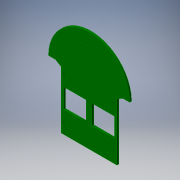
# Autodesk Inventor part: Micromouse1.2.kicad_pcb
Saved by Autodesk Inventor 2016 (Build 200138000, 138)
## iProperties
Created: 2017-09-20
Part Number: Micromouse1.2.kicad_pcb
Material: Generic
Document SubType Name: Modeling
Designer: test
Density: 1 g/cm^3
Appearance: Board Outline
Author: test
Autodesk Inventor part; units mm, degrees
ref_plane "YZ Plane" through (0, 0, 0) normal (1, 0, 0) x (0, 1, 0)
ref_plane "XZ Plane" through (0, 0, 0) normal (0, 1, 0) x (-1, 0, 0)
ref_plane "XY Plane" through (0, 0, 0) normal (0, 0, 1) x (1, 0, 0)
sketch "Sketch1" plane through (0, 0, 0) normal (0, 0, 1) x (1, 0, 0)
  line L0 (83.5624, -61.7466) -> (89.5624, -61.7716)
  line L1 (89.5624, -61.7716) -> (94.5924, -64.7466)
  line L2 (94.5924, -64.7466) -> (94.5924, -114.4666)
  line L3 (94.5924, -114.4666) -> (142.9124, -114.4666)
  line L4 (142.9124, -114.4666) -> (142.9124, -64.7466)
  line L5 (142.9124, -64.7466) -> (148.0124, -61.7466)
  line L6 (148.0124, -61.7466) -> (153.9624, -61.7466)
  arc A0 (153.9624, -61.7466) -> (83.5624, -61.7466) centre (118.7624, -61.7466) ccw
  line L7 (96.775, -95.75) -> (96.775, -78.75)
  line L8 (96.775, -78.75) -> (116.275, -78.75)
  line L9 (116.275, -78.75) -> (116.275, -95.75)
  line L10 (116.275, -95.75) -> (96.775, -95.75)
  line L11 (121.25, -95.775) -> (121.25, -78.775)
  line L12 (121.25, -78.775) -> (140.75, -78.775)
  line L13 (140.75, -78.775) -> (140.75, -95.775)
  line L14 (140.75, -95.775) -> (121.25, -95.775)
  line L15 (130.3424, -108.4516) -> (130.6424, -108.4516)
  arc A1 (130.6424, -109.0016) -> (130.6424, -108.4516) centre (130.6424, -108.7266) ccw
  line L16 (130.6424, -109.0016) -> (130.3424, -109.0016)
  arc A2 (130.3424, -108.4516) -> (130.3424, -109.0016) centre (130.3424, -108.7266) ccw
  line L17 (135.3424, -108.4516) -> (135.6424, -108.4516)
  arc A3 (135.6424, -109.0016) -> (135.6424, -108.4516) centre (135.6424, -108.7266) ccw
  line L18 (135.6424, -109.0016) -> (135.3424, -109.0016)
  arc A4 (135.3424, -108.4516) -> (135.3424, -109.0016) centre (135.3424, -108.7266) ccw
  line L19 (129.7424, -111.1016) -> (129.7424, -111.7516)
  arc A5 (129.2424, -111.7516) -> (129.7424, -111.7516) centre (129.4924, -111.7516) ccw
  line L20 (129.2424, -111.7516) -> (129.2424, -111.1016)
  arc A6 (129.7424, -111.1016) -> (129.2424, -111.1016) centre (129.4924, -111.1016) ccw
  line L21 (136.7424, -111.1016) -> (136.7424, -111.7516)
  arc A7 (136.2424, -111.7516) -> (136.7424, -111.7516) centre (136.4924, -111.7516) ccw
  line L22 (136.2424, -111.7516) -> (136.2424, -111.1016)
  arc A8 (136.7424, -111.1016) -> (136.2424, -111.1016) centre (136.4924, -111.1016) ccw
  circle A9 centre (88.0524, -59.1866) radius 0.45
  circle A10 centre (85.5195, -59.3771) radius 0.45
  circle A11 centre (112.8524, -37.2166) radius 0.45
  circle A12 centre (110.6984, -38.5626) radius 0.45
  circle A13 centre (127.4524, -38.4866) radius 0.45
  circle A14 centre (125.2984, -37.1406) radius 0.45
  circle A15 centre (129.9924, -44.7466) radius 0.45
  circle A16 centre (128.5355, -42.666) radius 0.45
  circle A17 centre (146.5124, -56.2766) radius 0.45
  circle A18 centre (143.9833, -56.042) radius 0.45
  circle A19 centre (117.3124, -33.4566) radius 0.45
  circle A20 centre (115.1584, -34.8026) radius 0.45
  circle A21 centre (105.3925, -47.0869) radius 0.45
  circle A22 centre (103.8924, -49.1366) radius 0.45
  circle A23 centre (133.2993, -49.4472) radius 0.45
  circle A24 centre (131.8424, -47.3666) radius 0.45
  circle A25 centre (122.9924, -34.4966) radius 0.45
  circle A26 centre (120.8384, -33.1506) radius 0.45
  circle A27 centre (151.7915, -59.8612) radius 0.45
  circle A28 centre (149.2624, -59.6266) radius 0.45
  circle A29 centre (93.5153, -55.9661) radius 0.45
  circle A30 centre (90.9824, -56.1566) radius 0.45
  circle A31 centre (108.6624, -42.1366) radius 0.45
  circle A32 centre (107.1623, -44.1863) radius 0.45
  circle A33 centre (25.5324, -58.5866) radius 0.5
  circle A34 centre (22.9924, -58.5866) radius 0.5
  circle A35 centre (20.4524, -58.5866) radius 0.5
  circle A36 centre (17.9124, -58.5866) radius 0.5
  circle A37 centre (108.7824, -100.5166) radius 0.5
  circle A38 centre (108.7824, -97.9766) radius 0.5
  circle A39 centre (106.2424, -100.5166) radius 0.5
  circle A40 centre (106.2424, -97.9766) radius 0.5
  circle A41 centre (103.7024, -100.5166) radius 0.5
  circle A42 centre (103.7024, -97.9766) radius 0.5
  circle A43 centre (97.2624, -105.2666) radius 1
  circle A44 centre (97.2624, -69.2666) radius 1
  circle A45 centre (117.6824, -75.6166) radius 0.45
  circle A46 centre (120.1824, -75.6166) radius 0.45
  circle A47 centre (121.7624, -124.4716) radius 0.381
  circle A48 centre (118.7624, -124.4716) radius 0.381
  circle A49 centre (115.7624, -124.4716) radius 0.381
  circle A50 centre (140.2874, -69.2666) radius 1
  circle A51 centre (140.2874, -105.2666) radius 1
  circle A52 centre (129.0424, -98.2966) radius 0.5
  circle A53 centre (129.0424, -100.8366) radius 0.5
  circle A54 centre (131.5824, -98.2966) radius 0.5
  circle A55 centre (131.5824, -100.8366) radius 0.5
  circle A56 centre (134.1224, -98.2966) radius 0.5
  circle A57 centre (134.1224, -100.8366) radius 0.5
  constraints: 58 centre point, 46 end point, 18 point on circle
extrude "Micromouse1.2.kicad_pcb_Outline" add sketch "Sketch1" along normal blind 1.6
sketch "Sketch2" plane through (25.5324, -58.5866, 1.6) normal (0, 0, 1) x (1, 0, 0)
  circle A0 centre (-7.62, 0) radius 0.5 projected
  circle A1 centre (-5.08, 0) radius 0.5 projected
  circle A2 centre (-2.54, 0) radius 0.5 projected
  circle A3 centre (0, 0) radius 0.5 projected
  circle A4 centre (90.23, -65.885) radius 0.381 projected
  circle A5 centre (93.23, -65.885) radius 0.381 projected
  circle A6 centre (96.23, -65.885) radius 0.381 projected
  point P0 (-25.5324, 58.5866)
extrude "Extrusion2" cut sketch "Sketch2" against normal through all
body "Solid1"
